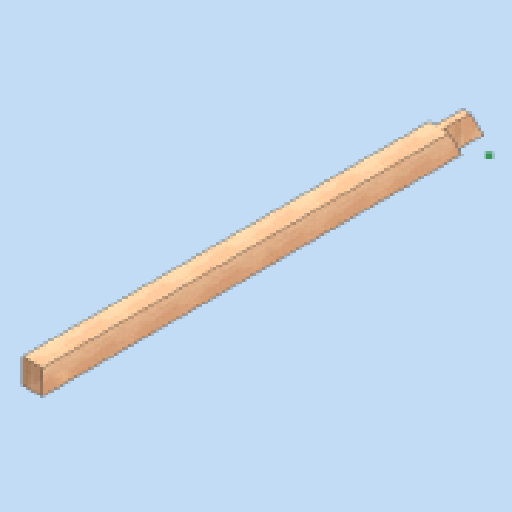
# Autodesk Inventor part: poutre100x80
Saved by Autodesk Inventor 2023 (Build 270158000, 158)
## iProperties
Created: 2026-03-19
Part Number: poutre100x80
Material: Wood (Birch)
Document SubType Name: Modeling
Designer: Nathann
Density: 0.55 g/cm^3
Appearance: Birch - Natural Polished
Mass: 6600 g
Surface Area: 5560 cm^2
Volume: 12000 cm^3
Author: Nathann
Autodesk Inventor part; units mm, degrees
ref_plane "YZ Plane" through (0, 0, 0) normal (1, 0, 0) x (0, 1, 0)
ref_plane "XZ Plane" through (0, 0, 0) normal (0, 1, 0) x (-1, 0, 0)
ref_plane "XY Plane" through (0, 0, 0) normal (0, 0, 1) x (1, 0, 0)
sketch "Sketch1" plane through (0, 0, 0) normal (0, 0, 1) x (1, 0, 0)
  line L0 (-40.3774, 59.0566) -> (39.6226, 59.0566)
  line L1 (39.6226, 59.0566) -> (39.6226, 159.0566)
  line L2 (39.6226, 159.0566) -> (-40.3774, 159.0566)
  line L3 (-40.3774, 159.0566) -> (-40.3774, 59.0566)
  point P0 (0, 0)
  dimension "d0" = 80
  dimension "d1" = 100
  constraints: 8 end point, 2 parallel, 1 horizontal, 1 perpendicular
  measures "d0" distance of L0.start L0.end
  measures "d1" distance of L2.end L0.start
extrude "Extrusion1" add sketch "Sketch1" along normal blind 1800
sketch "Sketch2" plane through (39.6226, 59.0566, 0) normal (1, 0, 0) x (0, 0, -1)
  line L0 (403.6788, -347.1669) -> (-104.7907, 650.76) projected
  line L1 (-104.7907, 650.76) -> (-128.8479, 638.5023) projected
  line L2 (379.6216, -359.4246) -> (-128.8479, 638.5023) projected
  line L3 (403.6788, -347.1669) -> (379.6216, -359.4246) projected
  line L4 (0, 0) -> (-1800, 0) projected
  line L5 (0, 0) -> (-117.0664, 229.7556)
  line L6 (-112.2326, 0) -> (-212.1687, 196.1355)
  line L7 (0, 0) -> (-112.2326, 0)
  line L8 (0, 0) -> (0, 100) projected
  line L9 (0, 100) -> (-1800, 100) projected
  line L10 (-163.1852, 100) -> (-50.9526, 100)
  point P0 (0, -59.0566)
  dimension "d4" = 100
  constraints: 8 end point, 5 point on line, 2 parallel, 1 perpendicular
  measures "d4" distance between parallel lines of L6 L5
extrude "Extrusion2" cut sketch "Sketch2" against normal blind 25 contours L4 L6 L9 L5
sketch "Sketch3" plane through (39.6226, 59.0566, 0) normal (1, 0, 0) x (0, 0, -1)
  line L0 (-50.9526, 100) -> (0, 0) projected
  line L1 (0, 0) -> (0, 100) projected
  line L2 (0, 100) -> (-50.9526, 100) projected
  point P0 (0, -59.0566)
sketch "Sketch4" plane through (39.6226, 59.0566, 0) normal (1, 0, 0) x (0, 0, -1)
  point P0 (0, -59.0566)
extrude "Extrusion3" cut sketch "Sketch3" against normal blind 100
sketch "Sketch5" plane through (-40.3774, 59.0566, 1800) normal (-1, 0, 0) x (0, 0, 1)
  line L0 (-1687.7674, 0) -> (-1636.8148, 100) projected
  line L1 (-1749.0474, 100) -> (-1800, 0) projected
  line L2 (-1800, 0) -> (0, 0) projected
  line L3 (0, 100) -> (0, 0) projected
  line L4 (-1749.0474, 100) -> (0, 100) projected
  point P0 (-1800, -59.0566)
  point P1 (-1687.7674, 0)
extrude "Extrusion4" cut sketch "Sketch5" against normal blind 25 contours L2 L1 L4 L0
body "Solid1"
